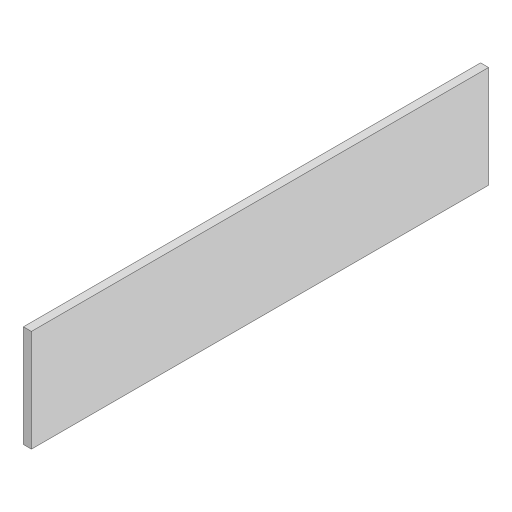
# Autodesk Inventor part: CUT PART O
Saved by Autodesk Inventor 2023.1 (Build 271208000, 208)
## iProperties
Created: 2022-11-08
Part Number: CUT PART O
Material: Generic
Document SubType Name: Modeling
Designer: GUT
Density: 1 g/cm^3
Appearance: Default
Author: GUT
Autodesk Inventor part; units mm, degrees
ref_plane "YZ Plane" through (0, 0, 0) normal (1, 0, 0) x (0, 1, 0)
ref_plane "XZ Plane" through (0, 0, 0) normal (0, 1, 0) x (-1, 0, 0)
ref_plane "XY Plane" through (0, 0, 0) normal (0, 0, 1) x (1, 0, 0)
sketch "Sketch1" plane through (0, 0, 0) normal (1, 0, 0) x (0, 1, 0)
  line L0 (-4.712, 16.0101) -> (148.288, 16.0101)
  line L1 (148.288, 16.0101) -> (148.288, -669.9899)
  line L2 (148.288, -669.9899) -> (-4.712, -669.9899)
  line L3 (-4.712, -669.9899) -> (-4.712, 16.0101)
  point P0 (0, 0)
  dimension "d0" = 153
  dimension "b" = 686
  constraints: 8 end point, 2 parallel, 1 horizontal, 1 perpendicular
  measures "d0" distance of L1.end L2.end
  measures "b" distance of L0.end L1.end
extrude "Extrusion1" add sketch "Sketch1" along normal blind 12
body "Solid1"
